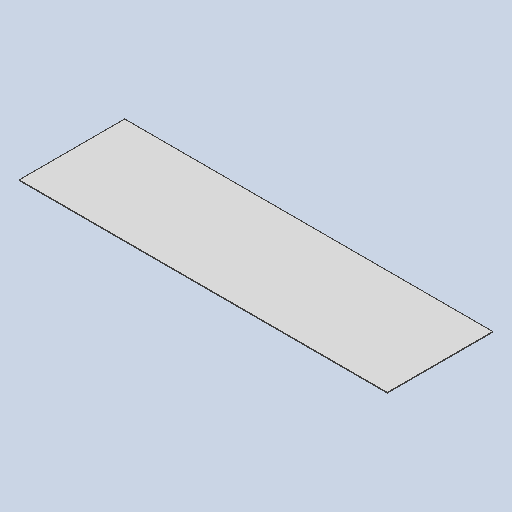
# Autodesk Inventor part: GBK bottom 0112
Saved by Autodesk Inventor 2026.2 (Build 302298000, 298)
## iProperties
Created: 2026-05-19
Part Number: GBK bottom 0112
Material: Steel
Document SubType Name: Sheet Metal
Designer: admin
Mass: 176625 g
Surface Area: 90450 cm^2
Volume: 22500 cm^3
Density: 7.85 g/cm^3
Flat Pattern Width: 85.4 cm
Flat Pattern Length: 298 cm
Flat Pattern Area: 25449.2 cm^2
Sheet Metal Rule: Default_mm
Sheet Metal Width: 854,000 mm
Sheet Metal Length: 2980,000 mm
Sheet Metal Area: 2544920,000 mm^2
Appearance: Default
Author: user
Autodesk Inventor part; units mm, degrees
ref_plane "YZ Plane" through (0, 0, 0) normal (1, 0, 0) x (0, 1, 0)
ref_plane "XZ Plane" through (0, 0, 0) normal (0, 1, 0) x (-1, 0, 0)
ref_plane "XY Plane" through (0, 0, 0) normal (0, 0, 1) x (1, 0, 0)
sketch "Эскиз1" plane through (0, 0, 0) normal (0, 1, 0) x (-1, 0, 0)
  line L0 (1490, 427) -> (-1490, 427)
  line L1 (-1490, 427) -> (-1490, -427)
  line L2 (-1490, -427) -> (1490, -427)
  line L3 (1490, -427) -> (1490, 427)
  line L4 (1490, 427) -> (-1490, -427) construction
  line L5 (-1490, 427) -> (1490, -427) construction
  point P0 (0, 0)
  dimension "d0" = 2980
  dimension "d1" = 854
  measures "d0" distance of L2.end L1.end
  measures "d1" distance of L1.end L0.end
extrude "Пластина1" add sketch "Эскиз1" along normal blind 5
equation "\"d2\" = Толщина"
equation "\"Радиус_гибки\" = Толщина"
equation "\"Ширина_просечки\" = Толщина"
equation "\"Глубина_просечки\" = 0.5 * Толщина"
equation "\"Радиус_перехода\" = Радиус_гибки"
equation "\"Радиус_Якоби\" = Радиус_гибки"
equation "\"Размер_зазора\" = Толщина"
equation "\"Толщина\" = 5"
